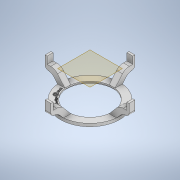
# Autodesk Inventor part: bottom part IKA adaptor
Saved by Autodesk Inventor 2022 (Build 260153000, 153)
## iProperties
Created: 2021-04-16
Part Number: bottom part IKA adaptor
Material: Generic
Document SubType Name: Modeling
Designer: tmass
Density: 1 g/cm^3
Appearance: Default
Author: tmass
Autodesk Inventor part; units mm, degrees
ref_plane "YZ Plane" through (0, 0, 0) normal (1, 0, 0) x (0, 1, 0)
sketch "Sketch1" plane through (0, 0, 0) normal (0, 1, 0) x (-1, 0, 0)
  circle A0 centre (0, 0) radius 40.025
  circle A1 centre (0, 0) radius 50.025
  dimension "d0" = 10
  dimension "d1" = 80.05
  constraints: 2 centre point, 2 coincident
  measures "d0" radial gap between concentric circles of A1 A0
  measures "d1" diameter of A0
extrude "Extrusion1" add sketch "Sketch1" along normal blind 5
ref_plane "Work Plane2" through (0, 5, 47.525) normal (0, 1, 0) x (1, 0, 0)
sketch "Sketch3" plane through (0, 5, 47.525) normal (0, 1, 0) x (1, 0, 0)
  circle A0 centre (0, 47.525) radius 40.1
  circle A1 centre (0, 47.525) radius 40.025 projected
  circle A2 centre (0, 47.525) radius 37.5
  dimension "d10" = 75
  dimension "d11" = 80.2
  constraints: 2 centre point, 2 coincident
  measures "d10" diameter of A2
  measures "d11" diameter of A0
extrude "Extrusion3" add sketch "Sketch3" against normal blind 2 contours A0 | A1
ref_plane "Work Plane3" through (0, 5, 47.525) normal (0, 1, 0) x (1, 0, 0)
sketch "Sketch4" plane through (0, 5, 47.525) normal (0, 1, 0) x (1, 0, 0)
  circle A0 centre (0, 47.525) radius 40.025 projected
  arc A1 (40.025, 47.5204) -> (-39.2567, 47.525) centre (0.3842, 47.6282) ccw
  line L0 (-8.8701, 5.9268) -> (-9.7228, 6.1468)
  line L1 (-9.7228, 6.1468) -> (-10.4153, 8.0687)
  line L2 (-10.4153, 8.0687) -> (-10.8371, 6.4343)
  line L3 (-10.8371, 6.4343) -> (-11.6983, 6.6566)
  line L4 (-11.6983, 6.6566) -> (-10.9362, 9.6098)
  line L5 (-10.9362, 9.6098) -> (-10.075, 9.3876)
  line L6 (-10.075, 9.3876) -> (-9.386, 7.4757)
  line L7 (-9.386, 7.4757) -> (-8.9664, 9.1015)
  line L8 (-8.9664, 9.1015) -> (-8.108, 8.88)
  line L9 (-8.108, 8.88) -> (-8.8701, 5.9268)
  line L10 (-11.5462, 9.8016) -> (-12.5608, 6.9253)
  line L11 (-12.5608, 6.9253) -> (-14.0418, 7.4477)
  spline S0 degree 2 poles (-14.0418, 7.4477) (-14.4515, 7.5922) (-14.8391, 7.8877) (-14.9701, 8.3635) (-14.8735, 8.6376) knots 0 0 0 1 2 3 3 3
  spline S1 degree 2 poles (-14.8735, 8.6376) (-14.7885, 8.8784) (-14.4616, 9.1522) (-14.2463, 9.1977) knots 0 0 0 1 2 2 2
  spline S2 degree 2 poles (-14.2463, 9.1977) (-14.1084, 9.2268) (-13.8935, 9.2008) knots 0 0 0 1 1 1
  spline S3 degree 2 poles (-13.8935, 9.2008) (-14.0327, 9.3091) (-14.0889, 9.388) knots 0 0 0 1 1 1
  spline S4 degree 2 poles (-14.0889, 9.388) (-14.1233, 9.4406) (-14.2267, 9.7386) (-14.2375, 9.814) knots 0 0 0 1 2 2 2
  line L12 (-14.2375, 9.814) -> (-14.3726, 10.7986)
  line L13 (-14.3726, 10.7986) -> (-13.3677, 10.4441)
  line L14 (-13.3677, 10.4441) -> (-13.2049, 9.3968)
  spline S5 degree 2 poles (-13.2049, 9.3968) (-13.1759, 9.1967) (-13.1252, 9.1197) knots 0 0 0 1 1 1
  spline S6 degree 2 poles (-13.1252, 9.1197) (-13.0517, 9.0191) (-12.9299, 8.9761) knots 0 0 0 1 1 1
  line L15 (-12.9299, 8.9761) -> (-12.8524, 8.9487)
  line L16 (-12.8524, 8.9487) -> (-12.4403, 10.117)
  line L17 (-12.4403, 10.117) -> (-11.5462, 9.8016)
  line L18 (-13.0438, 8.4062) -> (-13.4175, 8.538)
  spline S7 degree 2 poles (-13.4175, 8.538) (-13.4757, 8.5585) (-13.6638, 8.5813) knots 0 0 0 1 1 1
  spline S8 degree 2 poles (-13.6638, 8.5813) (-13.7592, 8.5931) (-13.9207, 8.4882) (-13.9539, 8.3941) knots 0 0 0 1 2 2 2
  spline S9 degree 2 poles (-13.9539, 8.3941) (-14.0027, 8.2557) (-13.8811, 8.0447) (-13.6374, 7.9588) knots 0 0 0 1 2 2 2
  line L19 (-13.6374, 7.9588) -> (-13.2499, 7.822)
  line L20 (-13.2499, 7.822) -> (-13.0438, 8.4062)
  line L21 (-16.5091, 10.5504) -> (-16.7709, 9.973)
  line L22 (-16.7709, 9.973) -> (-18.097, 10.5743)
  line L23 (-18.097, 10.5743) -> (-17.5612, 11.7559)
  spline S10 degree 2 poles (-17.5612, 11.7559) (-17.0601, 11.8446) (-16.3897, 11.7662) (-15.9887, 11.5844) knots 0 0 0 1 2 2 2
  spline S11 degree 2 poles (-15.9887, 11.5844) (-15.4941, 11.3601) (-15.0212, 10.7396) (-14.9821, 9.916) (-15.1785, 9.4829) knots 0 0 0 1 2 3 3 3
  spline S12 degree 2 poles (-15.1785, 9.4829) (-15.3846, 9.0284) (-16.0631, 8.5271) (-16.5067, 8.5155) knots 0 0 0 1 2 2 2
  spline S13 degree 2 poles (-16.5067, 8.5155) (-16.8508, 8.5104) (-17.3266, 8.7261) knots 0 0 0 1 1 1
  spline S14 degree 2 poles (-17.3266, 8.7261) (-17.7892, 8.9359) (-18.1712, 9.3089) (-18.3132, 9.7988) (-18.2669, 10.1001) knots 0 0 0 1 2 3 3 3
  line L24 (-18.2669, 10.1001) -> (-17.3702, 9.874)
  spline S15 degree 2 poles (-17.3702, 9.874) (-17.3909, 9.6932) (-17.2213, 9.4133) (-17.0315, 9.3272) knots 0 0 0 1 2 2 2
  spline S16 degree 2 poles (-17.0315, 9.3272) (-16.7508, 9.1999) (-16.2357, 9.4402) (-16.043, 9.8653) knots 0 0 0 1 2 2 2
  spline S17 degree 2 poles (-16.043, 9.8653) (-15.8393, 10.3144) (-16.0031, 10.856) (-16.3079, 10.9942) knots 0 0 0 1 2 2 2
  spline S18 degree 2 poles (-16.3079, 10.9942) (-16.4522, 11.0597) (-16.7518, 11.0956) (-16.9663, 11.0704) knots 0 0 0 1 2 2 2
  line L25 (-16.9663, 11.0704) -> (-17.0839, 10.8111)
  line L26 (-17.0839, 10.8111) -> (-16.5091, 10.5504)
  line L27 (-22.6368, 11.6574) -> (-21.063, 14.27)
  line L28 (-21.063, 14.27) -> (-20.3841, 13.861)
  line L29 (-20.3841, 13.861) -> (-20.5522, 13.5819)
  spline S19 degree 2 poles (-20.5522, 13.5819) (-20.3038, 13.6756) (-20.1493, 13.6647) knots 0 0 0 1 1 1
  spline S20 degree 2 poles (-20.1493, 13.6647) (-19.9409, 13.6523) (-19.7498, 13.5371) knots 0 0 0 1 1 1
  spline S21 degree 2 poles (-19.7498, 13.5371) (-19.3626, 13.3039) (-19.3097, 12.4701) (-19.5626, 12.0502) knots 0 0 0 1 2 2 2
  spline S22 degree 2 poles (-19.5626, 12.0502) (-19.8459, 11.58) (-20.5974, 11.3507) (-20.9444, 11.5597) knots 0 0 0 1 2 2 2
  spline S23 degree 2 poles (-20.9444, 11.5597) (-21.1154, 11.6627) (-21.3238, 11.9425) (-21.3598, 12.1218) knots 0 0 0 1 2 2 2
  line L30 (-21.3598, 12.1218) -> (-21.9051, 11.2166)
  line L31 (-21.9051, 11.2166) -> (-22.6368, 11.6574)
  spline S24 degree 2 poles (-20.9089, 12.8817) (-21.0437, 12.6579) (-20.9869, 12.3255) (-20.8435, 12.2392) knots 0 0 0 1 2 2 2
  spline S25 degree 2 poles (-20.8435, 12.2392) (-20.7178, 12.1635) (-20.4196, 12.2717) (-20.2711, 12.5181) knots 0 0 0 1 2 2 2
  spline S26 degree 2 poles (-20.2711, 12.5181) (-20.1318, 12.7494) (-20.1775, 13.0717) (-20.3083, 13.1505) knots 0 0 0 1 2 2 2
  spline S27 degree 2 poles (-20.3083, 13.1505) (-20.4466, 13.2338) (-20.7604, 13.1281) (-20.9089, 12.8817) knots 0 0 0 1 2 2 2
  line L32 (-24.0198, 15.2353) -> (-22.6329, 14.2579)
  spline S28 degree 2 poles (-22.6329, 14.2579) (-22.5337, 14.4394) (-22.5482, 14.5717) knots 0 0 0 1 1 1
  spline S29 degree 2 poles (-22.5482, 14.5717) (-22.5637, 14.7586) (-22.7269, 14.8736) knots 0 0 0 1 1 1
  spline S30 degree 2 poles (-22.7269, 14.8736) (-22.8277, 14.9446) (-22.9567, 14.9602) knots 0 0 0 1 1 1
  spline S31 degree 2 poles (-22.9567, 14.9602) (-23.0356, 14.9655) (-23.1579, 14.9295) knots 0 0 0 1 1 1
  line L33 (-23.1579, 14.9295) -> (-23.7954, 15.4722)
  spline S32 degree 2 poles (-23.7954, 15.4722) (-23.4483, 15.6334) (-22.837, 15.5581) (-22.4243, 15.2672) knots 0 0 0 1 2 2 2
  spline S33 degree 2 poles (-22.4243, 15.2672) (-22.0644, 15.0136) (-21.7961, 14.5229) (-21.8361, 13.8903) (-22.0458, 13.5927) knots 0 0 0 1 2 3 3 3
  spline S34 degree 2 poles (-22.0458, 13.5927) (-22.3451, 13.168) (-23.2561, 13.0271) (-23.7336, 13.3636) knots 0 0 0 1 2 2 2
  spline S35 degree 2 poles (-23.7336, 13.3636) (-24.1223, 13.6376) (-24.4053, 14.189) (-24.3259, 14.801) (-24.0756, 15.1561) knots 0 0 0 1 2 3 3 3
  line L34 (-24.0756, 15.1561) -> (-24.0198, 15.2353)
  spline S36 degree 2 poles (-23.5477, 14.407) (-23.6706, 14.1919) (-23.6171, 13.8957) (-23.4732, 13.7942) knots 0 0 0 1 2 2 2
  spline S37 degree 2 poles (-23.4732, 13.7942) (-23.31, 13.6792) (-23.1186, 13.7419) knots 0 0 0 1 1 1
  spline S38 degree 2 poles (-23.1186, 13.7419) (-22.9987, 13.7795) (-22.8686, 13.9284) knots 0 0 0 1 1 1
  line L35 (-22.8686, 13.9284) -> (-23.5477, 14.407)
  line L36 (-24.0809, 15.6388) -> (-24.7823, 16.1069)
  spline S39 degree 2 poles (-24.7823, 16.1069) (-24.7289, 16.2564) (-24.7932, 16.4752) (-24.9139, 16.5733) knots 0 0 0 1 2 2 2
  spline S40 degree 2 poles (-24.9139, 16.5733) (-25.0483, 16.6826) (-25.1675, 16.6849) knots 0 0 0 1 1 1
  spline S41 degree 2 poles (-25.1675, 16.6849) (-25.2578, 16.6902) (-25.3096, 16.6264) knots 0 0 0 1 1 1
  spline S42 degree 2 poles (-25.3096, 16.6264) (-25.367, 16.5558) (-25.3233, 16.456) knots 0 0 0 1 1 1
  spline S43 degree 2 poles (-25.3233, 16.456) (-25.2909, 16.3842) (-25.0965, 16.158) knots 0 0 0 1 1 1
  spline S44 degree 2 poles (-25.0965, 16.158) (-24.8007, 15.8192) (-24.6175, 15.5) (-24.6316, 15.1104) (-24.7575, 14.9555) knots 0 0 0 1 2 3 3 3
  spline S45 degree 2 poles (-24.7575, 14.9555) (-24.8945, 14.787) (-25.2927, 14.7021) (-25.7347, 14.861) (-26.0263, 15.098) knots 0 0 0 1 2 3 3 3
  spline S46 degree 2 poles (-26.0263, 15.098) (-26.3338, 15.348) (-26.5494, 15.6784) (-26.5861, 16.0336) (-26.5128, 16.254) knots 0 0 0 1 2 3 3 3
  line L37 (-26.5128, 16.254) -> (-25.8387, 15.8081)
  spline S47 degree 2 poles (-25.8387, 15.8081) (-25.8803, 15.7057) (-25.8571, 15.6225) knots 0 0 0 1 1 1
  spline S48 degree 2 poles (-25.8571, 15.6225) (-25.8223, 15.5072) (-25.7107, 15.4165) knots 0 0 0 1 1 1
  spline S49 degree 2 poles (-25.7107, 15.4165) (-25.6013, 15.3276) (-25.434, 15.324) (-25.3877, 15.3809) knots 0 0 0 1 2 2 2
  spline S50 degree 2 poles (-25.3877, 15.3809) (-25.3377, 15.4424) (-25.3779, 15.528) knots 0 0 0 1 1 1
  spline S51 degree 2 poles (-25.3779, 15.528) (-25.4139, 15.614) (-25.6099, 15.815) knots 0 0 0 1 1 1
  spline S52 degree 2 poles (-25.6099, 15.815) (-25.9082, 16.1181) (-26.122, 16.5113) (-26.0906, 16.8943) (-25.9721, 17.0401) knots 0 0 0 1 2 3 3 3
  spline S53 degree 2 poles (-25.9721, 17.0401) (-25.8498, 17.1904) (-25.4421, 17.3243) (-24.922, 17.1776) (-24.5895, 16.9073) knots 0 0 0 1 2 3 3 3
  spline S54 degree 2 poles (-24.5895, 16.9073) (-24.118, 16.524) (-23.9379, 15.9311) (-24.0809, 15.6388) knots 0 0 0 1 2 2 2
  line L38 (-27.3157, 16.2524) -> (-27.946, 16.8203)
  line L39 (-27.946, 16.8203) -> (-26.4664, 18.4625)
  line L40 (-26.4664, 18.4625) -> (-25.8361, 17.8946)
  line L41 (-25.8361, 17.8946) -> (-27.3157, 16.2524)
  line L42 (-27.8777, 15.6287) -> (-28.508, 16.1966)
  line L43 (-28.508, 16.1966) -> (-28.1229, 16.624)
  line L44 (-28.1229, 16.624) -> (-27.4926, 16.0561)
  line L45 (-27.4926, 16.0561) -> (-27.8777, 15.6287)
  line L46 (-29.5228, 18.3493) -> (-30.0823, 18.9107)
  line L47 (-30.0823, 18.9107) -> (-28.6039, 20.384)
  line L48 (-28.6039, 20.384) -> (-28.5373, 20.4544)
  spline S55 degree 2 poles (-28.5373, 20.4544) (-28.3897, 20.6015) (-27.9992, 20.742) (-27.6257, 20.6999) (-27.2338, 20.4522) (-27.0287, 20.2463) knots 0 0 0 1 2 3 4 4 4
  spline S56 degree 2 poles (-27.0287, 20.2463) (-26.5583, 19.7743) (-26.4909, 19.1411) (-26.7279, 18.9049) knots 0 0 0 1 2 2 2
  spline S57 degree 2 poles (-26.7279, 18.9049) (-26.757, 18.8759) (-26.809, 18.8282) knots 0 0 0 1 1 1
  line L49 (-26.809, 18.8282) -> (-27.3227, 19.4767)
  spline S58 degree 2 poles (-27.3227, 19.4767) (-27.2644, 19.5804) (-27.2808, 19.6552) knots 0 0 0 1 1 1
  spline S59 degree 2 poles (-27.2808, 19.6552) (-27.2993, 19.7652) (-27.3988, 19.865) knots 0 0 0 1 1 1
  spline S60 degree 2 poles (-27.3988, 19.865) (-27.5293, 19.996) (-27.793, 19.9861) (-27.9656, 19.8141) knots 0 0 0 1 2 2 2
  line L50 (-27.9656, 19.8141) -> (-28.2005, 19.58)
  spline S61 degree 2 poles (-28.2005, 19.58) (-28.0095, 19.5962) (-27.8726, 19.5545) knots 0 0 0 1 1 1
  spline S62 degree 2 poles (-27.8726, 19.5545) (-27.6631, 19.4898) (-27.5014, 19.3276) knots 0 0 0 1 1 1
  spline S63 degree 2 poles (-27.5014, 19.3276) (-27.1906, 19.0157) (-27.2724, 18.5488) knots 0 0 0 1 1 1
  spline S64 degree 2 poles (-27.2724, 18.5488) (-27.3311, 18.2168) (-27.6513, 17.8977) knots 0 0 0 1 1 1
  spline S65 degree 2 poles (-27.6513, 17.8977) (-28.0173, 17.533) (-28.7521, 17.5052) (-29.036, 17.7901) knots 0 0 0 1 2 2 2
  spline S66 degree 2 poles (-29.036, 17.7901) (-29.2183, 17.973) (-29.3298, 18.3344) (-29.292, 18.5793) knots 0 0 0 1 2 2 2
  line L51 (-29.292, 18.5793) -> (-29.5228, 18.3493)
  spline S67 degree 2 poles (-28.2023, 18.5421) (-28.0318, 18.712) (-28.0105, 19.0192) (-28.1286, 19.1377) knots 0 0 0 1 2 2 2
  spline S68 degree 2 poles (-28.1286, 19.1377) (-28.2385, 19.2479) (-28.5602, 19.2298) (-28.7307, 19.0599) knots 0 0 0 1 2 2 2
  spline S69 degree 2 poles (-28.7307, 19.0599) (-28.9033, 18.8879) (-28.9267, 18.5496) (-28.8128, 18.4352) knots 0 0 0 1 2 2 2
  spline S70 degree 2 poles (-28.8128, 18.4352) (-28.6988, 18.3209) (-28.3957, 18.3494) (-28.2023, 18.5421) knots 0 0 0 1 2 2 2
  line L52 (-30.5393, 19.4033) -> (-31.0552, 20.0011)
  line L53 (-31.0552, 20.0011) -> (-30.7818, 20.237)
  spline S71 degree 2 poles (-30.7818, 20.237) (-31.0658, 20.2246) (-31.4458, 20.3774) (-31.6146, 20.573) knots 0 0 0 1 2 2 2
  spline S72 degree 2 poles (-31.6146, 20.573) (-31.8447, 20.8397) (-31.7858, 21.414) (-31.4569, 21.6978) knots 0 0 0 1 2 2 2
  line L54 (-31.4569, 21.6978) -> (-30.3923, 22.6164)
  line L55 (-30.3923, 22.6164) -> (-29.8361, 21.9719)
  line L56 (-29.8361, 21.9719) -> (-30.7562, 21.178)
  spline S73 degree 2 poles (-30.7562, 21.178) (-30.914, 21.0418) (-30.9454, 20.8131) (-30.8534, 20.7064) knots 0 0 0 1 2 2 2
  spline S74 degree 2 poles (-30.8534, 20.7064) (-30.7537, 20.5908) (-30.4534, 20.5979) (-30.2245, 20.7954) knots 0 0 0 1 2 2 2
  line L57 (-30.2245, 20.7954) -> (-29.42, 21.4896)
  line L58 (-29.42, 21.4896) -> (-28.8658, 20.8473)
  line L59 (-28.8658, 20.8473) -> (-30.5393, 19.4033)
  line L60 (-38.1098, 25.4128) -> (-35.0521, 26.7144)
  spline S75 degree 2 poles (-35.0521, 26.7144) (-34.9582, 26.7525) (-34.9184, 26.7775) knots 0 0 0 1 1 1
  spline S76 degree 2 poles (-34.9184, 26.7775) (-34.8537, 26.8181) (-34.8278, 26.9314) (-34.8715, 27.001) knots 0 0 0 1 2 2 2
  spline S77 degree 2 poles (-34.8715, 27.001) (-34.9745, 27.1651) (-35.2466, 27.2785) knots 0 0 0 1 1 1
  spline S78 degree 2 poles (-35.2466, 27.2785) (-35.6458, 27.4508) (-36.6899, 27.3364) (-37.2568, 26.9806) knots 0 0 0 1 2 2 2
  spline S79 degree 2 poles (-37.2568, 26.9806) (-38.1868, 26.3971) (-38.5933, 24.6589) (-38.0285, 23.7587) knots 0 0 0 1 2 2 2
  spline S80 degree 2 poles (-38.0285, 23.7587) (-37.6135, 23.0973) (-36.2985, 22.4045) (-34.7218, 22.5759) (-33.9958, 23.0315) knots 0 0 0 1 2 3 3 3
  spline S81 degree 2 poles (-33.9958, 23.0315) (-32.8619, 23.7429) (-32.336, 25.8541) (-32.9725, 26.8687) knots 0 0 0 1 2 2 2
  spline S82 degree 2 poles (-32.9725, 26.8687) (-33.2814, 27.361) (-34.1838, 28.0701) (-34.7742, 28.2819) knots 0 0 0 1 2 2 2
  line L61 (-34.7742, 28.2819) -> (-35.2266, 29.003)
  spline S83 degree 2 poles (-35.2266, 29.003) (-34.7025, 28.9299) (-34.3431, 28.788) knots 0 0 0 1 1 1
  spline S84 degree 2 poles (-34.3431, 28.788) (-33.8194, 28.5829) (-32.8248, 27.7931) (-32.4566, 27.2063) knots 0 0 0 1 2 2 2
  spline S85 degree 2 poles (-32.4566, 27.2063) (-31.948, 26.3956) (-31.8895, 24.6233) (-32.8233, 23.0186) (-33.6637, 22.4912) knots 0 0 0 1 2 3 3 3
  spline S86 degree 2 poles (-33.6637, 22.4912) (-34.544, 21.9389) (-36.4605, 21.79) (-38.0158, 22.5676) (-38.5556, 23.428) knots 0 0 0 1 2 3 3 3
  spline S87 degree 2 poles (-38.5556, 23.428) (-39.2515, 24.537) (-38.7178, 26.8125) (-37.5988, 27.5146) knots 0 0 0 1 2 2 2
  spline S88 degree 2 poles (-37.5988, 27.5146) (-36.9374, 27.9296) (-35.4982, 28.0772) (-34.8491, 27.7497) knots 0 0 0 1 2 2 2
  spline S89 degree 2 poles (-34.8491, 27.7497) (-34.3477, 27.5029) (-34.1231, 27.1448) knots 0 0 0 1 1 1
  spline S90 degree 2 poles (-34.1231, 27.1448) (-33.992, 26.936) (-34.0224, 26.5426) (-34.1957, 26.3438) knots 0 0 0 1 2 2 2
  spline S91 degree 2 poles (-34.1957, 26.3438) (-33.8203, 26.2536) (-33.3879, 25.9842) (-33.2444, 25.7555) knots 0 0 0 1 2 2 2
  spline S92 degree 2 poles (-33.2444, 25.7555) (-32.9511, 25.288) (-33.3075, 24.1217) (-34.0386, 23.6631) knots 0 0 0 1 2 2 2
  spline S93 degree 2 poles (-34.0386, 23.6631) (-34.8989, 23.1232) (-36.8393, 23.1117) (-37.245, 23.7583) knots 0 0 0 1 2 2 2
  spline S94 degree 2 poles (-37.245, 23.7583) (-37.401, 24.0069) (-37.4075, 24.5365) (-37.2408, 24.9114) knots 0 0 0 1 2 2 2
  line L62 (-37.2408, 24.9114) -> (-37.6792, 24.7265)
  line L63 (-37.6792, 24.7265) -> (-38.1098, 25.4128)
  spline S95 degree 2 poles (-34.3344, 24.5101) (-33.9117, 24.7754) (-33.7953, 25.0979) knots 0 0 0 1 1 1
  spline S96 degree 2 poles (-33.7953, 25.0979) (-33.7054, 25.3414) (-33.8365, 25.5503) knots 0 0 0 1 1 1
  spline S97 degree 2 poles (-33.8365, 25.5503) (-33.9769, 25.7741) (-34.5908, 25.9018) (-35.9112, 25.4546) (-36.3687, 25.1675) knots 0 0 0 1 2 3 3 3
  spline S98 degree 2 poles (-36.3687, 25.1675) (-36.7119, 24.9522) (-36.8808, 24.4372) (-36.7529, 24.2333) knots 0 0 0 1 2 2 2
  spline S99 degree 2 poles (-36.7529, 24.2333) (-36.6063, 23.9996) (-36.3199, 23.9298) knots 0 0 0 1 1 1
  spline S100 degree 2 poles (-36.3199, 23.9298) (-35.9345, 23.8458) (-34.7571, 24.2449) (-34.3344, 24.5101) knots 0 0 0 1 2 2 2
  line L64 (-39.1437, 31.4929) -> (-39.5094, 32.3582)
  line L65 (-39.5094, 32.3582) -> (-37.8356, 33.0656)
  spline S101 degree 2 poles (-37.8356, 33.0656) (-37.5869, 33.1707) (-37.0783, 33.204) (-36.6079, 33.0108) (-36.4625, 32.8555) knots 0 0 0 1 2 3 3 3
  spline S102 degree 2 poles (-36.4625, 32.8555) (-36.2616, 32.6441) (-36.1108, 32.2872) knots 0 0 0 1 1 1
  spline S103 degree 2 poles (-36.1108, 32.2872) (-36.0239, 32.0817) (-35.8762, 31.5736) (-35.9082, 31.1745) (-36.1076, 30.7715) (-36.2547, 30.652) knots 0 0 0 1 2 3 4 4 4
  spline S104 degree 2 poles (-36.2547, 30.652) (-36.4881, 30.4577) (-36.6963, 30.3697) knots 0 0 0 1 1 1
  line L66 (-36.6963, 30.3697) -> (-38.37, 29.6624)
  line L67 (-38.37, 29.6624) -> (-38.7357, 30.5276)
  line L68 (-38.7357, 30.5276) -> (-37.0214, 31.2522)
  spline S105 degree 2 poles (-37.0214, 31.2522) (-36.7916, 31.3493) (-36.6406, 31.7159) (-36.7366, 31.943) knots 0 0 0 1 2 2 2
  spline S106 degree 2 poles (-36.7366, 31.943) (-36.8314, 32.1674) (-37.1942, 32.3169) (-37.4294, 32.2175) knots 0 0 0 1 2 2 2
  line L69 (-37.4294, 32.2175) -> (-39.1437, 31.4929)
  line L70 (-38.9025, 33.1442) -> (-39.1814, 33.9795)
  line L71 (-39.1814, 33.9795) -> (-37.9898, 34.8322)
  line L72 (-37.9898, 34.8322) -> (-39.4584, 34.8093)
  line L73 (-39.4584, 34.8093) -> (-39.7289, 35.6196)
  line L74 (-39.7289, 35.6196) -> (-37.3347, 35.4285)
  line L75 (-37.3347, 35.4285) -> (-37.0968, 34.7156)
  line L76 (-37.0968, 34.7156) -> (-38.9025, 33.1442)
  line L77 (-38.6681, 38.3069) -> (-38.4058, 37.268)
  line L78 (-38.4058, 37.268) -> (-37.8796, 37.2465)
  line L79 (-37.8796, 37.2465) -> (-37.6438, 36.313)
  line L80 (-37.6438, 36.313) -> (-40.882, 36.6789)
  line L81 (-40.882, 36.6789) -> (-41.1343, 37.6779)
  line L82 (-41.1343, 37.6779) -> (-38.4575, 39.5348)
  line L83 (-38.4575, 39.5348) -> (-38.216, 38.5785)
  line L84 (-38.216, 38.5785) -> (-38.6681, 38.3069)
  line L85 (-39.2604, 37.9544) -> (-40.24, 37.3618)
  line L86 (-40.24, 37.3618) -> (-39.0965, 37.3055)
  line L87 (-39.0965, 37.3055) -> (-39.2604, 37.9544)
  constraints: 2 point on circle, 1 centre point, 3 other
emboss "Emboss1" sketch "Sketch4" operation add depth 1 direction (0, -1, 0) contours L9 L0 L1 L2 L3 L4 A0 L6 L7 | A0 L7 L8 L9 | L82 L83 L84 L77 L78 L79 L80 A0 | A0 L80 L81 L82 | A0 L4 L5 L6 | L74 L75 L76 A0 | A0 L76 L70 L71 L72 L73 L74 | L10 L11 S0 S1 S2 S3 S4 L12 A0 L14 S5 S6 L15 L16 | A0 L16 L17 L10 | S101 S102 S103 S104 A0 S105 S106 | A0 S106 L69 L64 L65 S101 | A0 L12 L13 L14 | A0 S104 L66 L67 L68 S105 | S11 S12 S13 S14 L24 S15 S16 S17 A0 | A0 S17 S18 L23 S10 S11 | S89 S90 A0 | A0 S90 S91 S92 S93 S94 L62 L63 L60 S75 S76 S77 S78 S79 S80 S81 S85 S86 S87 S88 S89 | S18 L25 L26 L21 L22 L23 A0 | S91 S92 A0 | S21 S22 S23 L30 L31 L27 A0 S27 S24 S25 S26 | A0 S26 S27 L27 L28 L29 S19 S20 S21 | S81 S82 L61 S83 S84 S85 A0 | L54 L55 L56 A0 | A0 L56 S73 S74 L57 L59 L52 L53 S71 S72 L54 | S33 S34 S35 L34 L32 S28 A0 | A0 S28 S29 S30 S31 L33 S32 S33 | L57 L58 L59 A0 | S42 S43 S44 S45 S46 L37 S47 S48 S49 S50 S51 S52 S53 A0 | A0 S53 S54 L36 S39 S40 S41 S42 | L47 L48 S55 S56 S57 L49 S58 S59 S60 L50 S61 S62 S63 S64 A0 S67 S68 | A0 S68 S69 S70 S67 S64 S65 S66 L51 L46 L47 | L41 L38 L39 A0 | A0 L39 L40 L41 | L42 L43 L44 L45
sketch "Sketch6" plane through (0, 0, 0) normal (1, 0, 0) x (0, 1, 0)
  line L0 (5, -50.025) -> (5, 50.025) projected
  line L1 (5, 0) -> (25, 0) construction
  line L2 (25, 128.4088) -> (25, -20.2694) construction
  line L3 (22, -71) -> (37, -71)
  line L4 (37, -71) -> (37, -66)
  line L5 (37, -66) -> (27, -66)
  line L6 (25, -64) -> (25, -61.3735)
  line L7 (5, -37.5) -> (19.6861, -49.9201)
  line L8 (17, -67.1328) -> (17, -66)
  line L9 (5, -50.025) -> (11.6861, -55.6795)
  arc A0 (17, -67.1328) -> (11.6861, -55.6795) centre (2, -67.1328) ccw
  arc A1 (25, -61.3735) -> (19.6861, -49.9201) centre (10, -61.3735) ccw
  arc A2 (25, -64) -> (27, -66) centre (27, -64) ccw
  arc A3 (17, -66) -> (22, -71) centre (22, -66) ccw
  point P0 (0, 0)
  point P1 (25, -66)
  point P2 (25, -54.4141)
  point P3 (17, -60.1735)
  dimension "d27" = 20
  dimension "d28" = 66
  dimension "d29" = 5
  dimension "d31" = 12
  dimension "d32" = 20
  dimension "d37" = 8
  dimension "d39" = 15
  dimension "d40" = 15
  dimension "d41" = 2
  dimension "d45" = 0
  dimension "d46" = 5
  constraints: 18 end point, 8 point on circle, 8 point on line, 8 tangent, 4 centre point, 3 perpendicular, 2 horizontal, 2 vertical, 1 coincident, 1 midpoint, 1 parallel
  measures "d27" distance of L1.start L1.end
  measures "d28" distance from line of point (25, 0) L5
  measures "d29" distance of L3.end L4.end
  measures "d31" distance of L4.end point (25, -66)
  measures "d32" distance between parallel lines of L0 L2
  measures "d37" distance between parallel lines of L6 L8
  measures "d39" radius of A0
  measures "d40" radius of A1
  measures "d41" radius of A2
  measures "d45" distance between parallel lines of L6 L2
  measures "d46" radius of A3
extrude "Extrusion4" add sketch "Sketch6" along normal mid plane 10
pattern_circular "Circular Pattern2" count 4 over 360 about axis through (0, -10, 0) along (0, 1, 0) of "Extrusion4"
ref_plane "Work Plane4" through (0, 25, 0) normal (0, 1, 0) x (1, 0, 0)
sketch "Sketch7" plane through (0, 25, 0) normal (0, 1, 0) x (1, 0, 0)
  circle A0 centre (0, 0) radius 67.5
  dimension "d48" = 135
  constraints: 1 centre point, 1 coincident
  measures "d48" diameter of A0
extrude "Extrusion5" cut sketch "Sketch7" along normal through all
body "Solid1"
